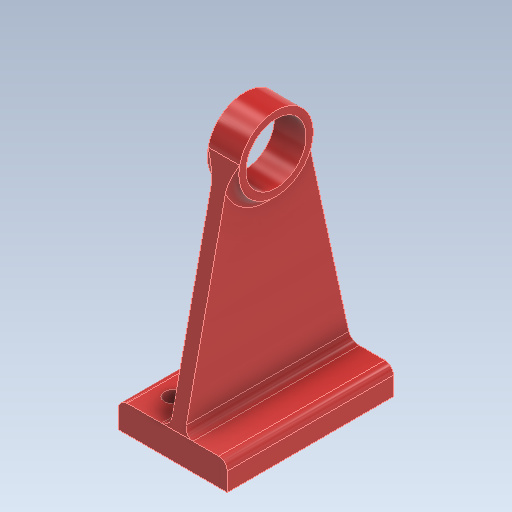
# Autodesk Inventor part: brackett
Saved by Autodesk Inventor 2021 (Build 250183000, 183)
## iProperties
Created: 2022-04-30
Part Number: brackett
Material: Generic
Document SubType Name: Modeling
Designer: authe
Density: 1 g/cm^3
Appearance: Orange-Red
Author: authe
Autodesk Inventor part; units mm, degrees
ref_plane "YZ Plane" through (0, 0, 0) normal (1, 0, 0) x (0, 1, 0)
ref_plane "XZ Plane" through (0, 0, 0) normal (0, 1, 0) x (-1, 0, 0)
ref_plane "XY Plane" through (0, 0, 0) normal (0, 0, 1) x (1, 0, 0)
sketch "Sketch1" plane through (0, 0, 0) normal (1, 0, 0) x (0, 1, 0)
  line L0 (0, 0) -> (9.5, 0)
  line L1 (9.5, 0) -> (9.5, -58)
  line L2 (9.5, -58) -> (0, -58)
  line L3 (0, -58) -> (0, 0)
  line L4 (0, 0) -> (0, -29)
  line L5 (0, -29) -> (82, -29)
  circle A0 centre (82, -29) radius 10.5
  circle A1 centre (82, -29) radius 13
  line L6 (84.7512, -16.2945) -> (9.5, 0)
  line L7 (84.7512, -41.7055) -> (9.5, -58)
  dimension "d2" = 9.5
  dimension "d3" = 58
  dimension "d4" = 29
  dimension "d5" = 82
  dimension "d6" = 21
  dimension "d7" = 26
  constraints: 16 end point, 2 centre point, 2 coincident, 2 parallel, 2 perpendicular, 2 point on circle, 2 tangent, 1 horizontal, 1 midpoint
  measures "d2" distance of L1.end L2.end
  measures "d3" distance of L0.end L1.end
  measures "d4" distance of L0.start L4.end
  measures "d5" distance of L4.end L5.end
  measures "d6" diameter of A0
  measures "d7" diameter of A1
extrude "Extrusion1" add sketch "Sketch1" along normal blind 5
extrude "Extrusion2" add sketch "Sketch1" along normal blind 8 and the other way blind 3 contours A1
extrude "Extrusion3" add sketch "Sketch1" along normal blind 20 and the other way blind 18 contours L0 L1 L5 L3 | L5 L1 L2 L3
fillet "Fillet1" radius 3 5 edges at (0, 9.5, -29) (-18, 9.5, -29) (20, 9.5, -29) (0, 69, -29) (5, 69, -29)
fillet "Fillet2" radius 3 1 edges at (5, 9.5, -29)
sketch "Sketch2" plane through (-18, 0, -58) normal (0, -1, 0) x (1, 0, 0)
  line L0 (0, 0) -> (0, 58) projected
  line L1 (0, 58) -> (0, 48)
  line L2 (0, 48) -> (9, 48)
  line L3 (0, 0) -> (0, 10)
  line L4 (0, 10) -> (9, 10)
  circle A0 centre (9, 48) radius 3
  circle A1 centre (9, 10) radius 3
  point P0 (18, 58)
  dimension "d20" = 10
  dimension "d21" = 9
  dimension "d22" = 10
  dimension "d23" = 9
  dimension "d24" = 6
  dimension "d25" = 6
  constraints: 8 end point, 2 centre point, 2 coincident, 2 perpendicular, 2 point on line
  measures "d20" distance of L0.end L1.end
  measures "d21" distance of L1.end L2.end
  measures "d22" distance of L0.start L3.end
  measures "d23" distance of L3.end L4.end
  measures "d24" diameter of A0
  measures "d25" diameter of A1
extrude "Extrusion4" cut sketch "Sketch2" against normal blind 20
body "Solid1"
